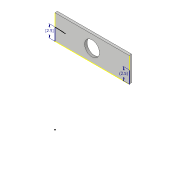
# Autodesk Inventor part: kj
Saved by Autodesk Inventor 2019 (Build 230136000, 136)
## iProperties
Created: 2019-11-13
Part Number: kj
Material: Generic
Document SubType Name: Modeling
Designer: Admin
Density: 1 g/cm^3
Appearance: Default
Author: Admin
Autodesk Inventor part; units mm, degrees
ref_plane "YZ Plane" through (0, 0, 0) normal (1, 0, 0) x (0, 1, 0)
ref_plane "XZ Plane" through (0, 0, 0) normal (0, 1, 0) x (-1, 0, 0)
ref_plane "XY Plane" through (0, 0, 0) normal (0, 0, 1) x (1, 0, 0)
sketch "Sketch1" plane through (0, 0, 0) normal (0, 0, 1) x (1, 0, 0)
  point P0 (0, 0)
sketch "Sketch2" plane through (0, 0, 0) normal (0, 0, 1) x (1, 0, 0)
  line L0 (0, 0) -> (150, 0)
  line L1 (150, 0) -> (150, 50)
  line L2 (150, 50) -> (0, 50)
  line L3 (0, 50) -> (0, 0)
  dimension "d0" = 150
  dimension "d1" = 50
  constraints: 8 end point, 2 parallel, 1 horizontal, 1 perpendicular
  measures "d0" distance of L2.end L1.end
  measures "d1" distance of L1.end L0.end
extrude "Extrusion1" add sketch "Sketch2" along normal blind 5
sketch "Sketch3" plane through (0, 0, 5) normal (0, 0, 1) x (1, 0, 0)
  line L0 (0, 0) -> (0, 25)
  line L1 (0, 50) -> (0, 0) projected
  arc A0 (20.6375, 23.8125) -> (0, 25) centre (0, -154.9228) ccw
  dimension "d4" = 25
  constraints: 2 end point, 2 point on circle, 1 centre point, 1 midpoint, 1 point on line
  measures "d4" distance of L0.start L0.end
sketch "Sketch4" plane through (0, 0, 5) normal (0, 0, 1) x (1, 0, 0)
  point P0 (0, 0)
sketch "Sketch5" plane through (0, 0, 5) normal (0, 0, 1) x (1, 0, 0)
  line L0 (0, 0) -> (150, 0) projected
  line L1 (150, 0) -> (150, 25)
  line L2 (150, 0) -> (150, 50) projected
  dimension "d5" = 25
  constraints: 2 end point, 1 midpoint
  measures "d5" distance of L0.end L1.end
sketch "Sketch6" plane through (0, 0, 5) normal (0, 0, 1) x (1, 0, 0)
  line L0 (150, 0) -> (150, 50) projected
  line L1 (150, 25) -> (90, 25)
  line L2 (90, 25) -> (60, 25)
  line L3 (60, 25) -> (0, 25)
  line L4 (0, 25) -> (75, 25)
  circle A0 centre (75, 25) radius 15
  point P0 (0, 0)
  dimension "d6" = 60
  dimension "d7" = 30
  dimension "d8" = 60
  dimension "d9" = 75
  dimension "d10" = 30
  constraints: 8 end point, 2 midpoint, 2 point on line, 1 centre point, 1 coincident, 1 horizontal
  measures "d6" distance of L1.start L1.end
  measures "d7" distance of L1.end L2.end
  measures "d8" distance of L2.end L3.end
  measures "d9" distance of L3.end L4.end
  measures "d10" diameter of A0
extrude "Extrusion2" cut sketch "Sketch6" against normal through all
body "Solid1"
